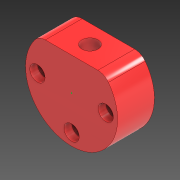
# Autodesk Inventor part: CH_01_0036_syringe_pump_mount
Saved by Autodesk Inventor 2022 (Build 260153000, 153)
## iProperties
Created: 2022-04-22
Part Number: CH_01_0036_syringe_pump_mount
Material: ABS Plastic
Document SubType Name: Modeling
Designer: Tomasz Krakowski
Density: 1.06 g/cm^3
Appearance: Light Red
Mass: 8.91114 g
Surface Area: 30.5837 cm^2
Volume: 8.40674 cm^3
Author: Tomasz Krakowski
Autodesk Inventor part; units mm, degrees
ref_plane "YZ Plane" through (0, 0, 0) normal (1, 0, 0) x (0, 1, 0)
ref_plane "XZ Plane" through (0, 0, 0) normal (0, 1, 0) x (-1, 0, 0)
ref_plane "XY Plane" through (0, 0, 0) normal (0, 0, 1) x (1, 0, 0)
sketch "Sketch1" plane through (0, 0, 0) normal (0, 0, 1) x (1, 0, 0)
  circle A0 centre (0, 0) radius 2
  arc A1 (-12.2474, 12.5) -> (12.2474, 12.5) centre (0, 0) ccw
  line L0 (-12.2474, 12.5) -> (12.2474, 12.5)
  dimension "d0" = 4
  dimension "d1" = 35
  dimension "d2" = 12.5
  constraints: 2 centre point, 2 coincident, 2 end point, 2 point on circle, 1 horizontal
  measures "d0" diameter of A0
  measures "d1" diameter of A1
  measures "d2" distance from line of L0 point (0, 0)
extrude "Extrusion1" add sketch "Sketch1" along normal blind 14
sketch "Sketch2" plane through (-12.2474, 12.5, 0) normal (0, 1, 0) x (1, 0, 0)
  line L0 (0, 0) -> (0, -14) construction
  line L1 (0, -7) -> (24.4949, -7) construction
  line L2 (24.4949, 0) -> (24.4949, -14) construction
  point P0 (12.2474, 0)
  point P1 (12.2474, -7)
  constraints: 3 midpoint, 2 end point
hole "Hole1" at (0, 12.5, 7) direction (0, -1, 0) diameter 6.2 depth 12.5 start extended yes
sketch "Sketch4" plane through (0, 0, 14) normal (0, 0, 1) x (1, 0, 0)
  circle A0 centre (0, 0) radius 2
  circle A1 centre (0, 0) radius 2 construction
  constraints: 1 centre point, 1 coincident, 1 concentric
extrude "Extrusion3" add sketch "Sketch4" against normal blind 5
sketch "Sketch5" plane through (0, 0, 14) normal (0, 0, 1) x (1, 0, 0)
  point P0 (0, 0)
sketch "Sketch6" plane through (0, 0, 0) normal (0, 0, -1) x (-1, 0, 0)
  circle A0 centre (0, 0) radius 4
  circle A1 centre (0, 0) radius 5.5
  dimension "d16" = 8
  dimension "d29" = 1.5
  constraints: 2 centre point, 2 coincident
  measures "d16" diameter of A0
  measures "d29" radial gap between concentric circles of A1 A0
extrude "Extrusion4" cut sketch "Sketch6" against normal blind 0.5
fillet "Fillet1" radius 0.5 2 edges at (4, 0, 0.5) (5.5, 0, 0.5)
fillet "Fillet2" radius 5 2 edges at (-12.2474, 12.5, 7) (12.2474, 12.5, 7)
sketch "Sketch8" plane through (0, 0, 14) normal (0, 0, 1) x (1, 0, 0)
  circle A0 centre (0, 0) radius 13 construction
  line L0 (-13, 0) -> (13, 0) construction
  line L1 (0, 0) -> (0, -13) construction
  dimension "d31" = 26
  constraints: 4 end point, 3 point on circle, 2 coincident, 1 centre point, 1 horizontal, 1 midpoint, 1 vertical
  measures "d31" diameter of A0
hole "Hole3" at (-13, 0, 14) at (13, 0, 14) at (0, -13, 14) direction (0, 0, -1) diameter 3.2 end through all counterbore diameter 5.8 counterbore depth 3
body "Solid1"
